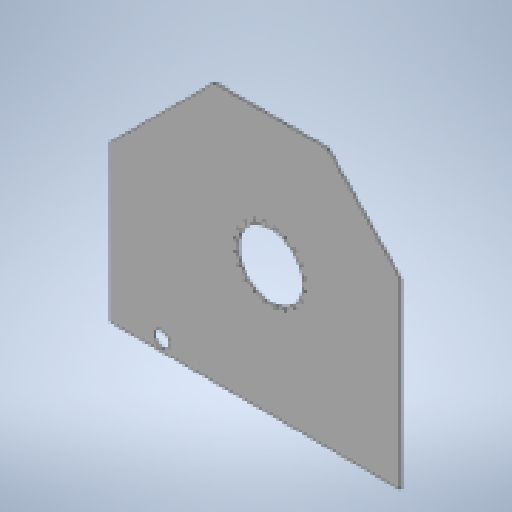
# Autodesk Inventor part: Wall right v2.0
Saved by Autodesk Inventor 2026.2 (Build 302298000, 298)
## iProperties
Created: 2023-08-31
Part Number: Wall right v2.0
Material: Generic
Document SubType Name: Sheet Metal
Designer: admin
Density: 1 g/cm^3
Appearance: Default
Flat Pattern Width: 191 cm
Flat Pattern Length: 214 cm
Flat Pattern Area: 40874 cm^2
Sheet Metal Rule: Default
Sheet Metal Width: 1910,000 mm
Sheet Metal Length: 2140,000 mm
Sheet Metal Area: 4087400,000 mm^2
Stock Number: ДМФ 010 Стенка_Корма
Author: admin
Autodesk Inventor part; units mm, degrees
ref_plane "YZ Plane" through (0, 0, 0) normal (1, 0, 0) x (0, 1, 0)
ref_plane "XZ Plane" through (0, 0, 0) normal (0, 1, 0) x (-1, 0, 0)
ref_plane "XY Plane" through (0, 0, 0) normal (0, 0, 1) x (1, 0, 0)
sketch "Sketch1" plane through (0, 0, 0) normal (0, 0, 1) x (1, 0, 0)
  line L0 (0, 0) -> (0, 1910) construction
  line L1 (424.5155, 1910) -> (-415.4845, 1910)
  line L2 (-415.4845, 1910) -> (-1180, 1150)
  line L3 (-1180, 0) -> (-1180, 1150)
  line L4 (960, 0) -> (960, 1342.8524)
  line L5 (424.5155, 1910) -> (960, 1342.8524)
  circle A0 centre (0, 950) radius 265 construction
  line L6 (960, 0) -> (-1180, 0)
  circle A1 centre (-1701.6377, -269.2167) radius 188.5 construction
  circle A2 centre (-800, 80) radius 55.5
  circle A3 centre (0, 950) radius 240
  line L7 (0, 1215) -> (0, 1190) construction
  circle A4 centre (51.6989, 1209.9081) radius 5.5
  line L8 (0, 950) -> (51.6989, 1209.9081) construction
  circle A5 centre (-51.6989, 1209.9081) radius 5.5
  circle A6 centre (-147.2261, 1170.3394) radius 5.5
  circle A7 centre (-220.3394, 1097.2261) radius 5.5
  circle A8 centre (-259.9081, 1001.6989) radius 5.5
  circle A9 centre (-259.9081, 898.3011) radius 5.5
  circle A10 centre (-220.3394, 802.7739) radius 5.5
  circle A11 centre (-147.2261, 729.6606) radius 5.5
  circle A12 centre (-51.6989, 690.0919) radius 5.5
  circle A13 centre (51.6989, 690.0919) radius 5.5
  circle A14 centre (147.2261, 729.6606) radius 5.5
  circle A15 centre (220.3394, 802.7739) radius 5.5
  circle A16 centre (259.9081, 898.3011) radius 5.5
  circle A17 centre (259.9081, 1001.6989) radius 5.5
  circle A18 centre (220.3394, 1097.2261) radius 5.5
  circle A19 centre (147.2261, 1170.3394) radius 5.5
  dimension "d72" = 480
  dimension "d1" = 840
  dimension "d3" = 1150
  dimension "d12" = 1180
  dimension "d13" = 950
  dimension "d14" = 111
  dimension "d15" = 1910
  dimension "d17" = -521.6377
  dimension "d18" = 377
  dimension "d19" = -269.2167
  dimension "d34" = 380
  dimension "d35" = 80
  dimension "d37" = 2140
  dimension "d52" = 530
  dimension "d69" = 780
  dimension "d71" = 1078
  dimension "d74" = 11
  dimension "d79" = 11.25
  dimension "d82" = 360
  constraints: 19 centre point, 18 end point, 17 coincident, 5 point on line, 3 vertical, 2 horizontal, 2 point on circle, 1 vertical alignment, 51 other
  measures "d1" distance of L1.start L1.end
  measures "d3" distance of L3.start L2.end
  measures "d12" distance from line of L3 A0.centre
  measures "d13" distance from line of L6 A0.centre
  measures "d14" diameter of A2
  measures "d15" vertical distance of L3.start L1.end
  measures "d17" distance from line of L3 A1.centre
  measures "d18" diameter of A1
  measures "d19" distance from line of A1.centre L6
  measures "d34" distance from line of A2.centre L3
  measures "d35" distance from line of A2.centre L6
  measures "d37" distance between parallel lines of L4 L3
  measures "d52" diameter of A0
  measures "d69" distance of L1.start L4.end
  measures "d71" distance of L1.end L2.end
  measures "d74" diameter of A4
  measures "d79" angle of L0 L8
extrude "Extrusion1" add sketch "Sketch1" along normal blind 10
fillet "Fillet1" [suppressed]
sketch "Sketch4" plane through (0, 0, 0) normal (0, 0, 1) x (1, 0, 0)
  circle A0 centre (-51.6989, 1209.9081) radius 6.5
  circle A1 centre (0, 950) radius 240 projected
  line L0 (0, 950) -> (0, 1196.7062) construction
  line L1 (-51.6989, 1209.9081) -> (0, 950) construction
  point P0 (0, 0)
  point P1 (240, 950)
  point P2 (-5, 1149.9375)
  point P3 (-2.5, 1189.987)
  point P4 (-168.8194, 970)
  point P5 (-2.5, 710.013)
  dimension "d59" = 265
  dimension "d60" = 13
  dimension "d61" = 11.25
  constraints: 4 end point, 1 centre point, 1 vertical
  measures "d59" distance of L0.start L1.start
  measures "d60" diameter of A0
  measures "d61" angle of L1 L0
extrude "Extrusion4" [suppressed]
pattern_circular "Circular Pattern3" [suppressed]
body "Solid1"
